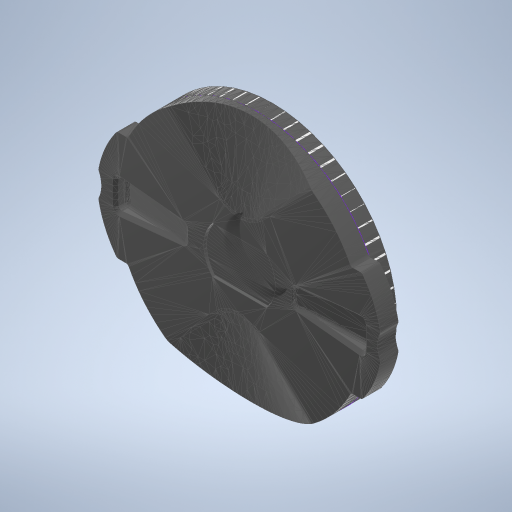
# Autodesk Inventor part: GarminQuarterTurn
Saved by Autodesk Inventor 2023 (Build 270158000, 158)
## iProperties
Created: 2022-10-27
Part Number: GarminQuarterTurn
Material: ABS Plastic
Document SubType Name: Modeling
Designer: jeron
Density: 1.06 g/cm^3
Appearance: Smooth - White
Author: jeron
Autodesk Inventor part; units mm, degrees
ref_plane "YZ Plane" through (0, 0, 0) normal (1, 0, 0) x (0, 1, 0)
ref_plane "XZ Plane" through (0, 0, 0) normal (0, 1, 0) x (-1, 0, 0)
ref_plane "Work Plane2" through (-56.0324, -131.572, 113.5507) normal (0, 0, 1) x (1, 0, 0)
sketch "Sketch2" plane through (-56.0324, -131.572, 113.5507) normal (0, 0, 1) x (1, 0, 0)
  circle A0 centre (56.0324, 131.572) radius 317.4946
  constraints: 1 centre point, 1 coincident
extrude "Extrusion1" add sketch "Sketch2" against normal blind 38.1
sketch "Sketch3" plane through (0, 0, 75.4507) normal (0, 0, -1) x (-1, 0, 0)
  circle A0 centre (0, 0) radius 84.3249
  constraints: 1 centre point, 1 coincident
extrude "Extrusion2" cut sketch "Sketch3" along normal mid plane 254
body "Solid1"
